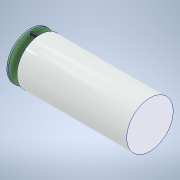
# Autodesk Inventor part: STACK NEW.
Saved by Autodesk Inventor 2021 (Build 250183000, 183)
## iProperties
Created: 2021-07-10
Part Number: STACK NEW.
Material: Glass
Document SubType Name: Modeling
Designer: HP
Density: 2.18 g/cm^3
Appearance: Cool White
Author: HP
Autodesk Inventor part; units mm, degrees
ref_plane "YZ Plane" through (0, 0, 0) normal (1, 0, 0) x (0, 1, 0)
ref_plane "XZ Plane" through (0, 0, 0) normal (0, 1, 0) x (-1, 0, 0)
ref_plane "XY Plane" through (0, 0, 0) normal (0, 0, 1) x (1, 0, 0)
sketch "Sketch1" plane through (0, 0, 0) normal (1, 0, 0) x (0, 1, 0)
  circle A0 centre (0, 0) radius 17.4625
  constraints: 1 centre point, 1 coincident
extrude "Extrusion1" add sketch "Sketch1" along normal blind 1.27
sketch "Sketch2" plane through (1.27, 0, 0) normal (1, 0, 0) x (0, 0, -1)
  circle A0 centre (0, 15.168) radius 1.27
  circle A1 centre (0, -14.7346) radius 1.27
  point P0 (0, 0)
  constraints: 2 centre point
extrude "Extrusion2" add sketch "Sketch2" along normal blind 88.9
sketch "Sketch3" plane through (90.17, 15.168, 0) normal (1, 0, 0) x (0, 0, -1)
  circle A0 centre (0, -15.168) radius 17.4625
  constraints: 1 centre point, 1 coincident
extrude "Extrusion3" add sketch "Sketch3" against normal blind 82.55
sketch "Sketch4" plane through (1.27, 0, 0) normal (1, 0, 0) x (0, 0, -1)
  point P0 (0, 0)
sketch "Sketch5" plane through (1.27, 0, 0) normal (1, 0, 0) x (0, 0, -1)
  point P0 (0, 0)
extrude "Extrusion4" [suppressed]
body "Solid1"
